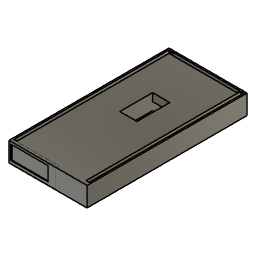
Top Plate (Autodesk Fusion 360 design; units mm, degrees)
Autodesk Fusion 360 part; units mm, degrees
sketch "Sketch1" plane through (0, 0, 0) normal (0, 0, 1) x (1, 0, 0)
  line L0 (-50, 100) -> (0, 100)
  line L1 (0, 100) -> (0, -2.5)
  line L2 (0, -2.5) -> (-50, -2.5)
  line L3 (-50, -2.5) -> (-50, 100)
  dimension "d1" = 50
  dimension "d2" = 102.5
  constraint horizontal L0
  constraint vertical L1
  constraint horizontal L2
  constraint vertical L3
  measures "d1" distance of L0.start L0.end
  measures "d2" distance of L0.start L2.end
extrude "Extrude1" add sketch "Sketch1" along normal blind 12.5
sketch "Sketch2" plane through (0, 0, 12.5) normal (0, 0, 1) x (-1, 0, 0)
  line L0 (50, 2.5) -> (0, 2.5)
  line L1 (0, 2.5) -> (0, -100)
  line L2 (0, -100) -> (50, -100)
  line L3 (50, -100) -> (50, 2.5)
  line L4 (50, -100) -> (49, -100)
  line L5 (49, -100) -> (49, -99)
  line L6 (49, -99) -> (47, -99)
  line L7 (47, -99) -> (47, 0)
  line L8 (47, 0) -> (49, 0)
  line L9 (49, 0) -> (49, -99)
  line L10 (50, -100) -> (0, -100)
  line L11 (3, -99) -> (3, 0)
  line L12 (1, 0) -> (1, -99)
  line L13 (1, -99) -> (3, -99)
  line L14 (3, 0) -> (1, 0)
  line L15 (47, -99) -> (46.5, -99)
  line L16 (46.5, -99) -> (3.5, -99)
  line L17 (3.5, -99) -> (3.5, -97)
  line L18 (3.5, -97) -> (46.5, -97)
  line L19 (46.5, -97) -> (46.5, -99)
  dimension "d5" = 2
  dimension "d6" = 99
  dimension "d7" = 43
  dimension "d8" = 2
  constraint coincident L2.end L3.start
  constraint coincident L2 L4.end
  constraint perpendicular L3 L4
  constraint perpendicular L4 L5
  constraint horizontal L6
  constraint vertical L7
  constraint horizontal L8
  constraint vertical L9
  constraint coincident L1.end L2.start
  constraint perpendicular L7 L15
  constraint horizontal L16
  constraint vertical L17
  constraint horizontal L18
  constraint vertical L19
  measures "d5" distance of L5.end L6.end
  measures "d6" distance of L5.end L8.end
  measures "d7" distance of L15.end L16.end
  measures "d8" distance of L15.end L18.end
extrude "Extrude2" cut sketch "Sketch2" against normal blind 3 contours L6 L7 L8 L9 | L11 L12 L13 L14 | L16 L17 L18 L19
sketch "Sketch3" plane through (0, 0, 12.5) normal (0, 0, 1) x (-1, 0, 0)
  line L0 (47, -99) -> (47, 0)
  line L1 (47, 0) -> (49, 0)
  line L2 (49, 0) -> (49, -99)
  line L3 (49, -99) -> (47, -99)
  line L4 (1, -99) -> (1, 0)
  line L5 (1, 0) -> (3, 0)
  line L6 (3, 0) -> (3, -99)
  line L7 (3, -99) -> (1, -99)
  line L8 (3.5, -99) -> (3.5, -97)
  line L9 (3.5, -97) -> (46.5, -97)
  line L10 (46.5, -97) -> (46.5, -99)
  line L11 (46.5, -99) -> (3.5, -99)
  line L12 (50, 2.5) -> (0, 2.5)
  line L13 (0, 2.5) -> (0, -100)
  line L14 (0, -100) -> (50, -100)
  line L15 (50, -100) -> (50, 2.5)
  line L16 (50, -100) -> (50, -70)
  line L17 (50, -70) -> (30.5, -70)
  line L18 (30.5, -70) -> (19.5, -70)
  line L19 (19.5, -70) -> (19.5, -49)
  line L20 (19.5, -49) -> (30.5, -49)
  line L21 (30.5, -49) -> (30.5, -70)
  dimension "d11" = 30
  dimension "d12" = 19.5
  dimension "d13" = 11
  dimension "d14" = 21
  constraint coincident L14.end L15.start
  constraint perpendicular L14 L16
  constraint perpendicular L0 L17
  constraint horizontal L18
  constraint vertical L19
  constraint horizontal L20
  constraint vertical L21
  measures "d11" distance of L14.end L16.end
  measures "d12" distance of L16.end L17.end
  measures "d13" distance of L17.end L18.end
  measures "d14" distance of L17.end L20.end
extrude "Extrude3" cut sketch "Sketch3" against normal blind 10 contours L18 L19 L20 L21
sketch "Sketch4" plane through (0, 0, 2.5) normal (0, 0, 1) x (-1, 0, 0)
  line L0 (30.5, -49) -> (19.5, -49)
  line L1 (19.5, -49) -> (19.5, -70)
  line L2 (19.5, -70) -> (30.5, -70)
  line L3 (30.5, -70) -> (30.5, -49)
  line L4 (30.5, -67.3616) -> (19.5, -67.3616)
  line L5 (19.5, -67.3616) -> (19.5, -100.8789)
  line L6 (19.5, -100.8789) -> (30.5, -100.8789)
  line L7 (30.5, -100.8789) -> (30.5, -67.3616)
  constraint horizontal L4
  constraint vertical L5
  constraint horizontal L6
  constraint vertical L7
  constraint coincident L3 L4.start
extrude "Extrude4" cut sketch "Sketch4" against normal blind 30 contours L2 L5 L6 L7
extrude "Extrude5" cut 1 faces at (-26.8333, 90, 2.5) along direction (0, 0, 1) blind 5
sketch "Sketch5" plane through (-50, 0, 0) normal (-1, 0, 0) x (0, -1, 0)
  line L0 (-100, 0) -> (2.5, 0)
  line L1 (2.5, 0) -> (2.5, 12.5)
  line L2 (2.5, 12.5) -> (-100, 12.5)
  line L3 (-100, 12.5) -> (-100, 0)
  line L4 (2.5, 0) -> (2.5, 2)
  line L5 (2.5, 2) -> (2, 2)
  line L6 (2, 2) -> (2, 11)
  line L7 (2, 11) -> (2.5, 11)
  line L8 (2, 11) -> (2, 12)
  line L9 (2, 12) -> (0.5, 12)
  line L10 (0.5, 12) -> (0.5, 0.4)
  line L11 (0.5, 0.4) -> (2, 0.4)
  line L12 (2, 0.4) -> (2, 2)
  dimension "d21" = 1.5
  dimension "d22" = 11.6
  constraint coincident L0.end L1.start
  constraint coincident L1 L4.end
  constraint perpendicular L1 L5
  constraint perpendicular L5 L6
  constraint coincident L1 L7.end
  constraint perpendicular L1 L7
  constraint perpendicular L7 L8
  constraint perpendicular L8 L9
  constraint perpendicular L9 L10
  constraint perpendicular L6 L11
  constraint perpendicular L5 L12
  measures "d21" distance of L8.end L9.end
  measures "d22" distance of L9.end L10.end
extrude "Extrude6" cut sketch "Sketch5" against normal blind 30 contours L6 L8 L9 L10 L11 L12
extrude "Extrude7" cut sketch "Sketch5" against normal blind 25 contours L1 L5 L6 L7
extrude "Extrude8" add sketch "Sketch5" against normal blind 1 contours L1 L5 L6 L7
